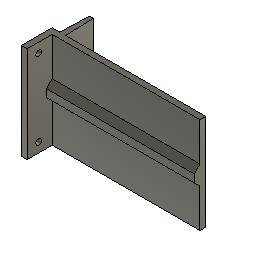
Holder_Bolts (Autodesk Fusion 360 design; units mm, degrees)
Autodesk Fusion 360 part; units mm, degrees
sketch "Skizze1" plane through (0, 0, 0) normal (0, 0, 1) x (1, 0, 0)
  line L0 (10, 10) -> (13, 10)
  line L1 (13, 10) -> (13, 23)
  line L2 (13, 23) -> (10, 23)
  line L3 (10, 23) -> (10, 10)
  line L4 (10, 23) -> (90, 23)
  line L5 (90, 23) -> (90, 26)
  line L6 (90, 26) -> (10, 26)
  line L7 (10, 26) -> (10, 23)
  line L8 (14, 26) -> (17, 26)
  line L9 (15.5, 26) -> (15.5, 41)
  line L10 (15.5, 41) -> (16.5, 41)
  line L11 (15.5, 41) -> (14.5, 41)
  line L12 (14.5, 41) -> (14, 26)
  line L13 (16.5, 41) -> (17, 26)
  dimension "d1" = 3
  dimension "d2" = 13
  dimension "d3" = 80
  dimension "d4" = 3
  dimension "d5" = 3
  dimension "d6" = 15
  dimension "d7" = 1
  dimension "d8" = 1
  measures "d3" distance of origin
extrude "Extrusion1" add sketch "Skizze1" along normal blind 50
sketch "Skizze2" plane through (13, 0, 0) normal (1, 0, 0) x (0, 1, 0)
  line L0 (10, 0) -> (23, 0)
  line L1 (23, 0) -> (23, 50)
  line L2 (23, 50) -> (10, 50)
  line L3 (10, 50) -> (10, 0)
  circle A0 centre (16, 45) radius 1.5
  circle A1 centre (16, 5) radius 1.5
  dimension "d11" = 3
  dimension "d12" = 3
  measures "d11" diameter of A0
  measures "d12" diameter of A1
extrude "Extrusion2" cut sketch "Skizze2" against normal blind 3 contours A0 | A1
sketch "Skizze3" plane through (0, 23, 0) normal (0, -1, 0) x (1, 0, 0)
  line L0 (13, 0) -> (90, 0)
  line L1 (90, 0) -> (90, 50)
  line L2 (90, 50) -> (13, 50)
  line L3 (13, 50) -> (13, 0)
  line L4 (90, 23) -> (13, 23)
  line L5 (13, 23) -> (13, 27)
  line L6 (13, 27) -> (90, 27)
  line L7 (90, 27) -> (90, 23)
  line L8 (90, 23) -> (13, 27) construction
  line L9 (13, 23) -> (90, 27) construction
  dimension "d15" = 4
extrude "Extrusion3" add sketch "Skizze3" along normal blind 3 contours L1 L3 L4 L5 L6 L7
chamfer "Fase1" distance 3 angle 45 1 edges at (51.5, 23, 27)
chamfer "Fase2" distance 3 angle 45 1 edges at (51.5, 23, 23)
